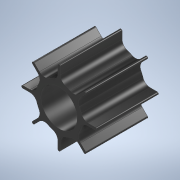
# Autodesk Inventor part: Valvula V2
Saved by Autodesk Inventor 2022 (Build 260153000, 153)
## iProperties
Created: 2021-02-16
Part Number: Valvula V2
Material: Generic
Document SubType Name: Modeling
Designer: juanp
Density: 1 g/cm^3
Appearance: Glossy - Black
Author: juanp
Autodesk Inventor part; units mm, degrees
ref_plane "YZ Plane" through (0, 0, 0) normal (1, 0, 0) x (0, 1, 0)
ref_plane "XZ Plane" through (0, 0, 0) normal (0, 1, 0) x (-1, 0, 0)
ref_plane "XY Plane" through (0, 0, 0) normal (0, 0, 1) x (1, 0, 0)
sketch "Sketch1" plane through (0, 0, 0) normal (0, 0, 1) x (1, 0, 0)
  circle A0 centre (0, 0) radius 7.5
  circle A1 centre (0, 0) radius 9.5
  line L0 (9.4868, 0.5) -> (15, 0.5)
  line L1 (9.4868, -0.5) -> (15, -0.5)
  arc A2 (15, -0.5) -> (15, 0.5) centre (15, 0) ccw
  line L2 (0, 0) -> (15, 0) construction
  line L3 (6.3547, 7.0618) -> (10.253, 10.9602)
  arc A3 (10.9602, 10.253) -> (10.253, 10.9602) centre (10.6066, 10.6066) ccw
  line L4 (7.0618, 6.3547) -> (10.9602, 10.253)
  line L5 (-0.5, 9.4868) -> (-0.5, 15)
  arc A4 (0.5, 15) -> (-0.5, 15) centre (0, 15) ccw
  line L6 (0.5, 9.4868) -> (0.5, 15)
  line L7 (-7.0618, 6.3547) -> (-10.9602, 10.253)
  arc A5 (-10.253, 10.9602) -> (-10.9602, 10.253) centre (-10.6066, 10.6066) ccw
  line L8 (-6.3547, 7.0618) -> (-10.253, 10.9602)
  line L9 (-9.4868, -0.5) -> (-15, -0.5)
  arc A6 (-15, 0.5) -> (-15, -0.5) centre (-15, 0) ccw
  line L10 (-9.4868, 0.5) -> (-15, 0.5)
  circle A7 centre (0, 0) radius 15.5 construction
  line L11 (-6.3547, -7.0618) -> (-10.253, -10.9602)
  arc A8 (-10.9602, -10.253) -> (-10.253, -10.9602) centre (-10.6066, -10.6066) ccw
  line L12 (-7.0618, -6.3547) -> (-10.9602, -10.253)
  line L13 (0.5, -9.4868) -> (0.5, -15)
  arc A9 (-0.5, -15) -> (0.5, -15) centre (0, -15) ccw
  line L14 (-0.5, -9.4868) -> (-0.5, -15)
  line L15 (7.0618, -6.3547) -> (10.9602, -10.253)
  arc A10 (10.253, -10.9602) -> (10.9602, -10.253) centre (10.6066, -10.6066) ccw
  line L16 (6.3547, -7.0618) -> (10.253, -10.9602)
  point P0 (-7.0618, 6.3547)
  point P1 (7.0618, 6.3547)
  point P2 (6.3547, 7.0618)
  point P3 (-6.3547, 7.0618)
  point P4 (-6.3547, -7.0618)
  point P5 (-7.0618, -6.3547)
  point P6 (7.0618, -6.3547)
  point P7 (0.5, -9.4868)
  dimension "d1" = 2
  dimension "d2" = 1
  dimension "d5" = 15
  dimension "d8" = 360
  dimension "d13" = 31
  dimension "d15" = 15
  constraints: 34 end point, 18 point on circle, 11 centre point, 3 coincident, 3 horizontal, 3 tangent, 65 other
  measures "d1" radial gap between concentric circles of A1 A0
  measures "d2" distance between parallel lines of L0 L1
  measures "d5" distance of point (0, 0) L2.end
  measures "d13" diameter of A7
  measures "d15" diameter of A0
extrude "Extrusion1" add sketch "Sketch1" along normal blind 25.5
fillet "Fillet1" radius 3 16 edges at (9.4868, 0.5, 12.75) (7.0618, 6.3547, 12.75) (-0.5, 9.4868, 12.75) (9.4868, -0.5, 12.75) (-9.4868, 0.5, 12.75) (-9.4868, -0.5, 12.75) (-7.0618, 6.3547, 12.75) (-6.3547, 7.0618, 12.75) (0.5, 9.4868, 12.75) (6.3547, 7.0618, 12.75) (-6.3547, -7.0618, 12.75) (-7.0618, -6.3547, 12.75) (-0.5, -9.4868, 12.75) (0.5, -9.4868, 12.75) (6.3547, -7.0618, 12.75) (7.0618, -6.3547, 12.75)
body "Solid1"
